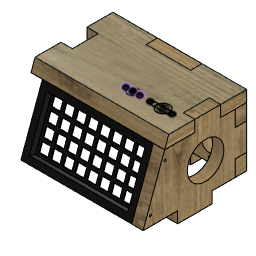
soundboard (Autodesk Fusion 360 design; units mm, degrees)
Autodesk Fusion 360 part; units mm, degrees
note: some values were not read from the file. Chosen so that the rebuilt part matches the saved one: which face or edge a step refers to. Set by a fixed rule: which sketch regions a step uses.
(part 1 of 2)
sketch "Skizze1" plane through (0, 0, 0) normal (1, 0, 0) x (0, 1, 0)
  line L0 (65, 65) -> (-65, 65)
  line L1 (-65, 65) -> (-65, -65)
  line L2 (-65, -65) -> (65, -65)
  line L3 (65, -65) -> (65, 65)
  line L4 (65, 65) -> (-65, -65) construction
  line L5 (-65, 65) -> (65, -65) construction
  circle A0 centre (0, 0) radius 29
  line L6 (65, 47) -> (-65, 47)
  line L7 (-65, -65) -> (-138, -65)
  line L8 (65, -47) -> (-138, -47)
  line L9 (-65, 47) -> (-99.2132, -47)
  line L10 (-65, 47) -> (35.0327, 47) construction
  line L11 (-99.2132, -47) -> (-99.2132, -65)
  line L12 (47, 65) -> (47, -65)
  dimension "d3" = 130
  dimension "d4" = 130
  dimension "d5" = 58
  dimension "d6" = 18
  dimension "d7" = 18
  dimension "d8" = 110
  dimension "d9" = 18
  constraint horizontal L0
  constraint perpendicular L0 L1
  constraint parallel L0 L2
  constraint parallel L1 L3
  constraint coincident L4 A0.centre
  constraint coincident L5 A0.centre
  constraint coincident A0.centre origin
  constraint coincident L3 L6.start
  constraint coincident L1 L6.end
  constraint perpendicular L1 L6
  constraint perpendicular L1 L7
  constraint coincident L3 L8.start
  constraint perpendicular L3 L8
  constraint horizontal L10
  constraint coincident L8 L9.end
  constraint coincident L7 L11.end
  constraint perpendicular L7 L11
  constraint coincident L0 L12.start
  constraint coincident L2 L12.end
  constraint perpendicular L2 L12
  measures "d3" distance of L1.end L2.end
  measures "d4" distance of L0.end L1.end
  measures "d5" diameter of A0
  measures "d6" distance of L0 L6
  measures "d7" distance of L7 L8
  measures "d8" angle of L9 L10
  measures "d9" distance of L3 L12
extrude "Extrusion1" add sketch "Skizze1" along normal blind 18 makes body 1
extrude "Extrusion2" add sketch "Skizze1" along normal blind 212.2 separate body contours L2 L3 L8 L12 | L1 L2 L8 L12 | L1 L7 L8 L11 makes body 2
extrude "Extrusion3" add sketch "Skizze1" along normal up to surface (212.2 mm away) separate body contours L0 L3 L6 L12 | L3 L6 L8 L12 | L2 L3 L8 L12 makes body 3
extrude "Extrusion4" add sketch "Skizze1" along normal up to surface (212.2 mm away) separate body contours L0 L3 L6 L12 | L0 L1 L6 L12 makes body 4
ref_plane "Arbeitsebene1" through (106.1, 0, 56) normal (1, 0, 0) x (0, 0, -1)
mirror "Spiegeln1" about plane through (106.1, 0, 56) normal (1, 0, 0) of bodies 1 makes body 5
ref_plane "Arbeitsebene2" through (18, -65, 47) normal (0, 0.939693, -0.34202) x (-1, 0, 0)
sketch "Skizze2" plane through (18, -65, 47) normal (0, 0.939693, -0.34202) x (-1, 0, 0)
  line L0 (18, 0) -> (-194.2, 0)
  line L1 (0, 0) -> (0, -100.0327)
  line L2 (18, -100.0327) -> (-194.2, -100.0327)
  line L3 (-176.2, 0) -> (-176.2, -100.0327)
  line L4 (18, -0.2) -> (-194.2, -0.2)
  line L5 (18, -99.8327) -> (-194.2, -99.8327)
  line L6 (-0.2, 0) -> (-0.2, -100.0327)
  line L7 (-176, 0) -> (-176, -100.0327)
  dimension "d22" = -0.2
  dimension "d23" = 0.2
  dimension "d24" = 0.2
  dimension "d25" = -0.2
ref_plane "Arbeitsebene3" through (106.1, -17.1066, 0) normal (-1, 0, 0) x (0, 1, 0)
sketch "Skizze3" plane through (106.1, -17.1066, 0) normal (-1, 0, 0) x (0, 1, 0)
  line L0 (-47.8934, -47) -> (-82.1066, 47)
  line L1 (-65, 0) -> (-52.8684, 0)
  line L2 (-65, 0) -> (-54.2875, 3.899) construction
  line L3 (-54.2875, 3.899) -> (-51.4492, -3.899) construction
  dimension "d73" = 11.4
  dimension "d74" = 12.1316
  dimension "d75" = 20
  dimension "d77" = 11.4
  constraint midpoint L0 L1.start
  constraint horizontal L1
  constraint perpendicular L0 L2
  constraint perpendicular L2 L3
  constraint midpoint L1.end L3
  measures "d73" distance of L1.start L2.end
  measures "d74" distance of L1.start L1.end
  measures "d75" angle of L1 L2
  measures "d77" distance of L1.start L2.end
sweep "Sweeping1" add profiles "Skizze2" path "Skizze3" along L1 section 1 contours L4 L5 L6 L7 separate body makes body 6
sketch "Skizze4" plane through (18, -65, 47) normal (0, 0.939693, -0.34202) x (-1, 0, 0)
  line L0 (-0.2, -0.2) -> (-0.2, -99.8327)
  line L1 (-0.2, -99.8327) -> (-176, -99.8327)
  line L2 (-176, -0.2) -> (-0.2, -0.2)
  line L3 (-14.6, -14.5158) -> (-28.6, -14.5158)
  line L4 (-28.6, -14.5158) -> (-28.6, -28.5158)
  line L5 (-28.6, -28.5158) -> (-14.6, -28.5158)
  line L6 (-14.6, -28.5158) -> (-14.6, -14.5158)
  line L7 (-33.6, -14.5158) -> (-47.6, -14.5158)
  line L8 (-33.6, -28.5158) -> (-33.6, -14.5158)
  line L9 (-47.6, -28.5158) -> (-33.6, -28.5158)
  line L10 (-47.6, -14.5158) -> (-47.6, -28.5158)
  line L11 (-52.6, -14.5158) -> (-66.6, -14.5158)
  line L12 (-52.6, -28.5158) -> (-52.6, -14.5158)
  line L13 (-66.6, -28.5158) -> (-52.6, -28.5158)
  line L14 (-66.6, -14.5158) -> (-66.6, -28.5158)
  line L15 (-71.6, -14.5158) -> (-85.6, -14.5158)
  line L16 (-71.6, -28.5158) -> (-71.6, -14.5158)
  line L17 (-85.6, -28.5158) -> (-71.6, -28.5158)
  line L18 (-85.6, -14.5158) -> (-85.6, -28.5158)
  line L19 (-90.6, -14.5158) -> (-104.6, -14.5158)
  line L20 (-90.6, -28.5158) -> (-90.6, -14.5158)
  line L21 (-104.6, -28.5158) -> (-90.6, -28.5158)
  line L22 (-104.6, -14.5158) -> (-104.6, -28.5158)
  line L23 (-109.6, -14.5158) -> (-123.6, -14.5158)
  line L24 (-109.6, -28.5158) -> (-109.6, -14.5158)
  line L25 (-123.6, -28.5158) -> (-109.6, -28.5158)
  line L26 (-123.6, -14.5158) -> (-123.6, -28.5158)
  line L27 (-128.6, -14.5158) -> (-142.6, -14.5158)
  line L28 (-128.6, -28.5158) -> (-128.6, -14.5158)
  line L29 (-142.6, -28.5158) -> (-128.6, -28.5158)
  line L30 (-142.6, -14.5158) -> (-142.6, -28.5158)
  line L31 (-147.6, -14.5158) -> (-161.6, -14.5158)
  line L32 (-147.6, -28.5158) -> (-147.6, -14.5158)
  line L33 (-161.6, -28.5158) -> (-147.6, -28.5158)
  line L34 (-161.6, -14.5158) -> (-161.6, -28.5158)
  line L35 (-14.6, -33.5158) -> (-28.6, -33.5158)
  line L36 (-14.6, -47.5158) -> (-14.6, -33.5158)
  line L37 (-28.6, -47.5158) -> (-14.6, -47.5158)
  line L38 (-28.6, -33.5158) -> (-28.6, -47.5158)
  line L39 (-33.6, -33.5158) -> (-47.6, -33.5158)
  line L40 (-33.6, -47.5158) -> (-33.6, -33.5158)
  line L41 (-47.6, -47.5158) -> (-33.6, -47.5158)
  line L42 (-47.6, -33.5158) -> (-47.6, -47.5158)
  line L43 (-52.6, -33.5158) -> (-66.6, -33.5158)
  line L44 (-52.6, -47.5158) -> (-52.6, -33.5158)
  line L45 (-66.6, -47.5158) -> (-52.6, -47.5158)
  line L46 (-66.6, -33.5158) -> (-66.6, -47.5158)
  line L47 (-71.6, -33.5158) -> (-85.6, -33.5158)
  line L48 (-71.6, -47.5158) -> (-71.6, -33.5158)
  line L49 (-85.6, -47.5158) -> (-71.6, -47.5158)
  line L50 (-85.6, -33.5158) -> (-85.6, -47.5158)
  line L51 (-90.6, -33.5158) -> (-104.6, -33.5158)
  line L52 (-90.6, -47.5158) -> (-90.6, -33.5158)
  line L53 (-104.6, -47.5158) -> (-90.6, -47.5158)
  line L54 (-104.6, -33.5158) -> (-104.6, -47.5158)
  line L55 (-109.6, -33.5158) -> (-123.6, -33.5158)
  line L56 (-109.6, -47.5158) -> (-109.6, -33.5158)
  line L57 (-123.6, -47.5158) -> (-109.6, -47.5158)
  line L58 (-123.6, -33.5158) -> (-123.6, -47.5158)
  line L59 (-128.6, -33.5158) -> (-142.6, -33.5158)
  line L60 (-128.6, -47.5158) -> (-128.6, -33.5158)
  line L61 (-142.6, -47.5158) -> (-128.6, -47.5158)
  line L62 (-142.6, -33.5158) -> (-142.6, -47.5158)
  line L63 (-147.6, -33.5158) -> (-161.6, -33.5158)
  line L64 (-147.6, -47.5158) -> (-147.6, -33.5158)
  line L65 (-161.6, -47.5158) -> (-147.6, -47.5158)
  line L66 (-161.6, -33.5158) -> (-161.6, -47.5158)
  line L67 (-14.6, -52.5158) -> (-28.6, -52.5158)
  line L68 (-14.6, -66.5158) -> (-14.6, -52.5158)
  line L69 (-28.6, -66.5158) -> (-14.6, -66.5158)
  line L70 (-28.6, -52.5158) -> (-28.6, -66.5158)
  line L71 (-33.6, -52.5158) -> (-47.6, -52.5158)
  line L72 (-33.6, -66.5158) -> (-33.6, -52.5158)
  line L73 (-47.6, -66.5158) -> (-33.6, -66.5158)
  line L74 (-47.6, -52.5158) -> (-47.6, -66.5158)
  line L75 (-52.6, -52.5158) -> (-66.6, -52.5158)
  line L76 (-52.6, -66.5158) -> (-52.6, -52.5158)
  line L77 (-66.6, -66.5158) -> (-52.6, -66.5158)
  line L78 (-66.6, -52.5158) -> (-66.6, -66.5158)
  line L79 (-71.6, -52.5158) -> (-85.6, -52.5158)
  line L80 (-71.6, -66.5158) -> (-71.6, -52.5158)
  line L81 (-85.6, -66.5158) -> (-71.6, -66.5158)
  line L82 (-85.6, -52.5158) -> (-85.6, -66.5158)
  line L83 (-90.6, -52.5158) -> (-104.6, -52.5158)
  line L84 (-90.6, -66.5158) -> (-90.6, -52.5158)
  line L85 (-104.6, -66.5158) -> (-90.6, -66.5158)
  line L86 (-104.6, -52.5158) -> (-104.6, -66.5158)
  line L87 (-109.6, -52.5158) -> (-123.6, -52.5158)
  line L88 (-109.6, -66.5158) -> (-109.6, -52.5158)
  line L89 (-123.6, -66.5158) -> (-109.6, -66.5158)
  line L90 (-123.6, -52.5158) -> (-123.6, -66.5158)
  line L91 (-128.6, -52.5158) -> (-142.6, -52.5158)
  line L92 (-128.6, -66.5158) -> (-128.6, -52.5158)
  line L93 (-142.6, -66.5158) -> (-128.6, -66.5158)
  line L94 (-142.6, -52.5158) -> (-142.6, -66.5158)
  line L95 (-147.6, -52.5158) -> (-161.6, -52.5158)
  line L96 (-147.6, -66.5158) -> (-147.6, -52.5158)
  line L97 (-161.6, -66.5158) -> (-147.6, -66.5158)
  line L98 (-161.6, -52.5158) -> (-161.6, -66.5158)
  line L99 (-14.6, -71.5158) -> (-28.6, -71.5158)
  line L100 (-14.6, -85.5158) -> (-14.6, -71.5158)
  line L101 (-28.6, -85.5158) -> (-14.6, -85.5158)
  line L102 (-28.6, -71.5158) -> (-28.6, -85.5158)
  line L103 (-33.6, -71.5158) -> (-47.6, -71.5158)
  line L104 (-33.6, -85.5158) -> (-33.6, -71.5158)
  line L105 (-47.6, -85.5158) -> (-33.6, -85.5158)
  line L106 (-47.6, -71.5158) -> (-47.6, -85.5158)
  line L107 (-52.6, -71.5158) -> (-66.6, -71.5158)
  line L108 (-52.6, -85.5158) -> (-52.6, -71.5158)
  line L109 (-66.6, -85.5158) -> (-52.6, -85.5158)
  line L110 (-66.6, -71.5158) -> (-66.6, -85.5158)
  line L111 (-71.6, -71.5158) -> (-85.6, -71.5158)
  line L112 (-71.6, -85.5158) -> (-71.6, -71.5158)
  line L113 (-85.6, -85.5158) -> (-71.6, -85.5158)
  line L114 (-85.6, -71.5158) -> (-85.6, -85.5158)
  line L115 (-90.6, -71.5158) -> (-104.6, -71.5158)
  line L116 (-90.6, -85.5158) -> (-90.6, -71.5158)
  line L117 (-104.6, -85.5158) -> (-90.6, -85.5158)
  line L118 (-104.6, -71.5158) -> (-104.6, -85.5158)
  line L119 (-109.6, -71.5158) -> (-123.6, -71.5158)
  line L120 (-109.6, -85.5158) -> (-109.6, -71.5158)
  line L121 (-123.6, -85.5158) -> (-109.6, -85.5158)
  line L122 (-123.6, -71.5158) -> (-123.6, -85.5158)
  line L123 (-128.6, -71.5158) -> (-142.6, -71.5158)
  line L124 (-128.6, -85.5158) -> (-128.6, -71.5158)
  line L125 (-142.6, -85.5158) -> (-128.6, -85.5158)
  line L126 (-142.6, -71.5158) -> (-142.6, -85.5158)
  line L127 (-147.6, -71.5158) -> (-161.6, -71.5158)
  line L128 (-147.6, -85.5158) -> (-147.6, -71.5158)
  line L129 (-161.6, -85.5158) -> (-147.6, -85.5158)
  line L130 (-161.6, -71.5158) -> (-161.6, -85.5158)
  line L131 (-0.2, 0) -> (-0.2, -100.0327)
  line L132 (-161.6, -85.5158) -> (-14.6, -14.5158) construction
  line L133 (-161.6, -14.5158) -> (-14.6, -85.5158) construction
  line L134 (18, -99.8327) -> (-194.2, -99.8327)
  line L135 (18, -0.2) -> (-194.2, -0.2)
  line L136 (-10.2, -89.8327) -> (-166.2, -89.8327)
  line L137 (-166.2, -89.8327) -> (-166.2, -10.2)
  line L138 (-166.2, -10.2) -> (-10.2, -10.2)
  line L139 (-10.2, -10.2) -> (-10.2, -89.8327)
  line L140 (-176, -99.8327) -> (-176, -0.2)
  point P0 (-88.1, -0.2)
  point P1 (-176.2, -50.0158)
  point P2 (-88.1, -50.0158)
  dimension "d33" = 14
  dimension "d34" = 14
  dimension "d37" = -19
  dimension "d38" = -19
  dimension "d41" = 14.5
  dimension "d42" = 14.3164
  dimension "d43" = 14.3164
  dimension "d52" = 14.4
  constraint horizontal L3
  constraint vertical L4
  constraint horizontal L5
  constraint vertical L6
  constraint midpoint L2 P0
  constraint midpoint L133 P2
  constraint horizontal P1 P2
  constraint vertical P0 P2
  constraint parallel L1 L136
  constraint parallel L2 L138
  constraint parallel L0 L139
  measures "d33" distance of L3.start L3.end
  measures "d34" distance of L3.start L5.end
  measures "d52" distance of L34 L140
sketch "Skizze5" plane through (106.1, -17.1066, 0) normal (-1, 0, 0) x (0, 1, 0)
  line L0 (-65, 0) -> (-52.8684, 0)
  line L1 (-65, 0) -> (-54.3582, 0)
  line L2 (-54.2875, 3.899) -> (-51.4492, -3.899)
  line L3 (-65, 0) -> (-54.2875, 3.899)
  line L4 (-55.6031, 3.4202) -> (-65, 0)
  point P0 (-52.8684, 0)
  point P1 (-55.6031, 3.4202)
  dimension "d76" = 1.4
  dimension "d79" = 1.4
  constraint coincident L0.start L1.start
  constraint coincident L0 L1.end
  constraint parallel L0 L1
  constraint coincident L3 P1
  constraint coincident P1 L4.start
  measures "d76" distance of L1.end L2
  measures "d79" distance of L2.start P1
sweep "Sweeping3" cut kept parallel profiles "Skizze4" path "Skizze5" along L4 section 1 contours L3 L4 L5 L6 | L7 L8 L9 L10 | L11 L12 L13 L14 | L15 L16 L17 L18 | L19 L20 L21 L22 | L23 L24 L25 L26 | L27 L28 L29 L30 | L31 L32 L33 L34 | L35 L36 L37 L38 | L39 L40 L41 L42 | L43 L44 L45 L46 | L47 L48 L49 L50 | L51 L52 L53 L54 | L55 L56 L57 L58 | L59 L60 L61 L62 | L63 L64 L65 L66 | L67 L68 L69 L70 | L71 L72 L73 L74 | L75 L76 L77 L78 | L79 L80 L81 L82 | L83 L84 L85 L86 | L87 L88 L89 L90 | L91 L92 L93 L94 | L95 L96 L97 L98 | L99 L100 L101 L102 | L103 L104 L105 L106 | L107 L108 L109 L110 | L111 L112 L113 L114 | L115 L116 L117 L118 | L119 L120 L121 L122 | L123 L124 L125 L126 | L127 L128 L129 L130 | L136 L137 L138 L139 bodies 6
sketch "Skizze6" plane through (0, -63.105, 22.9684) normal (0, -0.939693, 0.34202) x (1, 0, 0)
  line L0 (184.2, 14.4704) -> (28.2, 14.4704)
  line L1 (28.2, 14.4704) -> (28.2, -65.1623)
  line L2 (28.2, -65.1623) -> (184.2, -65.1623)
  line L3 (184.2, -65.1623) -> (184.2, 14.4704)
  line L4 (165.6, -6.5816) -> (165.6, 7.4184)
  line L5 (165.6, 7.4184) -> (179.6, 7.4184)
  line L6 (179.6, 7.4184) -> (179.6, -6.5816)
  line L7 (179.6, -6.5816) -> (165.6, -6.5816)
  line L8 (165.6, -11.5816) -> (179.6, -11.5816)
  line L9 (165.6, -25.5816) -> (165.6, -11.5816)
  line L10 (179.6, -25.5816) -> (165.6, -25.5816)
  line L11 (179.6, -11.5816) -> (179.6, -25.5816)
  line L12 (165.6, -30.5816) -> (179.6, -30.5816)
  line L13 (165.6, -44.5816) -> (165.6, -30.5816)
  line L14 (179.6, -44.5816) -> (165.6, -44.5816)
  line L15 (179.6, -30.5816) -> (179.6, -44.5816)
  line L16 (165.6, -49.5816) -> (179.6, -49.5816)
  line L17 (165.6, -63.5816) -> (165.6, -49.5816)
  line L18 (179.6, -63.5816) -> (165.6, -63.5816)
  line L19 (179.6, -49.5816) -> (179.6, -63.5816)
  line L20 (146.6, 7.4184) -> (160.6, 7.4184)
  line L21 (146.6, -6.5816) -> (146.6, 7.4184)
  line L22 (160.6, -6.5816) -> (146.6, -6.5816)
  line L23 (160.6, 7.4184) -> (160.6, -6.5816)
  line L24 (146.6, -11.5816) -> (160.6, -11.5816)
  line L25 (146.6, -25.5816) -> (146.6, -11.5816)
  line L26 (160.6, -25.5816) -> (146.6, -25.5816)
  line L27 (160.6, -11.5816) -> (160.6, -25.5816)
  line L28 (146.6, -30.5816) -> (160.6, -30.5816)
  line L29 (146.6, -44.5816) -> (146.6, -30.5816)
  line L30 (160.6, -44.5816) -> (146.6, -44.5816)
  line L31 (160.6, -30.5816) -> (160.6, -44.5816)
  line L32 (146.6, -49.5816) -> (160.6, -49.5816)
  line L33 (146.6, -63.5816) -> (146.6, -49.5816)
  line L34 (160.6, -63.5816) -> (146.6, -63.5816)
  line L35 (160.6, -49.5816) -> (160.6, -63.5816)
  line L36 (141.6, -49.5816) -> (141.6, -63.5816)
  line L37 (127.6, -49.5816) -> (141.6, -49.5816)
  line L38 (127.6, -63.5816) -> (127.6, -49.5816)
  line L39 (141.6, -63.5816) -> (127.6, -63.5816)
  line L40 (127.6, -30.5816) -> (141.6, -30.5816)
  line L41 (127.6, -44.5816) -> (127.6, -30.5816)
  line L42 (141.6, -44.5816) -> (127.6, -44.5816)
  line L43 (141.6, -30.5816) -> (141.6, -44.5816)
  line L44 (141.6, -25.5816) -> (127.6, -25.5816)
  line L45 (141.6, -11.5816) -> (141.6, -25.5816)
  line L46 (127.6, -11.5816) -> (141.6, -11.5816)
  line L47 (127.6, -25.5816) -> (127.6, -11.5816)
  line L48 (141.6, 7.4184) -> (141.6, -6.5816)
  line L49 (127.6, 7.4184) -> (141.6, 7.4184)
  line L50 (127.6, -6.5816) -> (127.6, 7.4184)
  line L51 (141.6, -6.5816) -> (127.6, -6.5816)
  line L52 (122.6, -6.5816) -> (108.6, -6.5816)
  line L53 (108.6, -6.5816) -> (108.6, 7.4184)
  line L54 (108.6, 7.4184) -> (122.6, 7.4184)
  line L55 (122.6, 7.4184) -> (122.6, -6.5816)
  line L56 (89.6, 7.4184) -> (103.6, 7.4184)
  line L57 (89.6, -6.5816) -> (89.6, 7.4184)
  line L58 (103.6, -6.5816) -> (89.6, -6.5816)
  line L59 (103.6, 7.4184) -> (103.6, -6.5816)
  line L60 (103.6, -44.5816) -> (89.6, -44.5816)
  line L61 (89.6, -44.5816) -> (89.6, -30.5816)
  line L62 (89.6, -30.5816) -> (103.6, -30.5816)
  line L63 (103.6, -30.5816) -> (103.6, -44.5816)
  line L64 (103.6, -25.5816) -> (89.6, -25.5816)
  line L65 (89.6, -25.5816) -> (89.6, -11.5816)
  line L66 (89.6, -11.5816) -> (103.6, -11.5816)
  line L67 (103.6, -11.5816) -> (103.6, -25.5816)
  line L68 (108.6, -11.5816) -> (122.6, -11.5816)
  line L69 (108.6, -25.5816) -> (108.6, -11.5816)
  line L70 (122.6, -25.5816) -> (108.6, -25.5816)
  line L71 (122.6, -11.5816) -> (122.6, -25.5816)
  line L72 (122.6, -44.5816) -> (108.6, -44.5816)
  line L73 (108.6, -44.5816) -> (108.6, -30.5816)
  line L74 (108.6, -30.5816) -> (122.6, -30.5816)
  line L75 (108.6, -49.5816) -> (122.6, -49.5816)
  line L76 (108.6, -63.5816) -> (108.6, -49.5816)
  line L77 (122.6, -63.5816) -> (108.6, -63.5816)
  line L78 (122.6, -49.5816) -> (122.6, -63.5816)
  line L79 (89.6, -49.5816) -> (103.6, -49.5816)
  line L80 (89.6, -63.5816) -> (89.6, -49.5816)
  line L81 (103.6, -63.5816) -> (89.6, -63.5816)
  line L82 (103.6, -49.5816) -> (103.6, -63.5816)
  line L83 (70.6, -49.5816) -> (84.6, -49.5816)
  line L84 (70.6, -63.5816) -> (70.6, -49.5816)
  line L85 (84.6, -63.5816) -> (70.6, -63.5816)
  line L86 (84.6, -49.5816) -> (84.6, -63.5816)
  line L87 (84.6, -30.5816) -> (84.6, -44.5816)
  line L88 (70.6, -30.5816) -> (84.6, -30.5816)
  line L89 (70.6, -44.5816) -> (70.6, -30.5816)
  line L90 (84.6, -44.5816) -> (70.6, -44.5816)
  line L91 (70.6, -25.5816) -> (70.6, -11.5816)
  line L92 (70.6, -11.5816) -> (84.6, -11.5816)
  line L93 (84.6, -11.5816) -> (84.6, -25.5816)
  line L94 (84.6, -25.5816) -> (70.6, -25.5816)
  line L95 (70.6, -6.5816) -> (70.6, 7.4184)
  line L96 (70.6, 7.4184) -> (84.6, 7.4184)
  line L97 (84.6, 7.4184) -> (84.6, -6.5816)
  line L98 (84.6, -6.5816) -> (70.6, -6.5816)
  line L99 (51.6, 7.4184) -> (65.6, 7.4184)
  line L100 (51.6, -6.5816) -> (51.6, 7.4184)
  line L101 (65.6, -6.5816) -> (51.6, -6.5816)
  line L102 (65.6, 7.4184) -> (65.6, -6.5816)
  line L103 (51.6, -11.5816) -> (65.6, -11.5816)
  line L104 (51.6, -25.5816) -> (51.6, -11.5816)
  line L105 (65.6, -25.5816) -> (51.6, -25.5816)
  line L106 (65.6, -11.5816) -> (65.6, -25.5816)
  line L107 (51.6, -30.5816) -> (65.6, -30.5816)
  line L108 (51.6, -44.5816) -> (51.6, -30.5816)
  line L109 (65.6, -44.5816) -> (51.6, -44.5816)
  line L110 (65.6, -30.5816) -> (65.6, -44.5816)
  line L111 (51.6, -49.5816) -> (65.6, -49.5816)
  line L112 (51.6, -63.5816) -> (51.6, -49.5816)
  line L113 (65.6, -63.5816) -> (51.6, -63.5816)
  line L114 (65.6, -49.5816) -> (65.6, -63.5816)
  line L115 (32.6, 7.4184) -> (46.6, 7.4184)
  line L116 (32.6, -6.5816) -> (32.6, 7.4184)
  line L117 (46.6, -6.5816) -> (32.6, -6.5816)
  line L118 (46.6, 7.4184) -> (46.6, -6.5816)
  line L119 (32.6, -11.5816) -> (46.6, -11.5816)
  line L120 (32.6, -25.5816) -> (32.6, -11.5816)
  line L121 (46.6, -25.5816) -> (32.6, -25.5816)
  line L122 (46.6, -11.5816) -> (46.6, -25.5816)
  line L123 (32.6, -30.5816) -> (46.6, -30.5816)
  line L124 (32.6, -44.5816) -> (32.6, -30.5816)
  line L125 (46.6, -44.5816) -> (32.6, -44.5816)
  line L126 (46.6, -30.5816) -> (46.6, -44.5816)
  line L127 (32.6, -49.5816) -> (46.6, -49.5816)
  line L128 (32.6, -63.5816) -> (32.6, -49.5816)
  line L129 (46.6, -63.5816) -> (32.6, -63.5816)
  line L130 (46.6, -49.5816) -> (46.6, -63.5816)
  line L131 (122.6, -30.5816) -> (122.6, -44.5816)
  line L132 (28.2, 11.7342) -> (28.2, -67.8985)
  line L133 (28.2, -67.8985) -> (184.2, -67.8985)
  line L134 (184.2, -67.8985) -> (184.2, 11.7342)
  line L135 (184.2, 11.7342) -> (28.2, 11.7342)
  line L136 (184.2, 11.7342) -> (28.2, 11.7342)
  line L137 (28.2, 11.7342) -> (28.2, -67.8985)
  line L138 (28.2, -67.8985) -> (184.2, -67.8985)
  line L139 (184.2, -67.8985) -> (184.2, 11.7342)
extrude "Extrusion5" cut sketch "Skizze6" against normal up to surface (1.4 mm away) contours L4 L5 L6 L7 | L8 L9 L10 L11 | L12 L13 L14 L15 | L16 L17 L18 L19 | L20 L21 L22 L23 | L24 L25 L26 L27 | L28 L29 L30 L31 | L32 L33 L34 L35 | L36 L37 L38 L39 | L40 L41 L42 L43 | L44 L45 L46 L47 | L48 L49 L50 L51 | L52 L53 L54 L55 | L56 L57 L58 L59 | L60 L61 L62 L63 | L64 L65 L66 L67 | L68 L69 L70 L71 | L72 L73 L74 L131 | L75 L76 L77 L78 | L79 L80 L81 L82 | L83 L84 L85 L86 | L87 L88 L89 L90 | L91 L92 L93 L94 | L95 L96 L97 L98 | L99 L100 L101 L102 | L103 L104 L105 L106 | L107 L108 L109 L110 | L111 L112 L113 L114 | L115 L116 L117 L118 | L119 L120 L121 L122 | L123 L124 L125 L126 | L127 L128 L129 L130 bodies 6
sketch "Skizze7" plane through (0, 0, 0) normal (1, 0, 0) x (0, 1, 0)
  line L0 (-65, 47) -> (-99.2132, -47)
  line L1 (-65, 65) -> (65, 65)
  line L2 (65, 65) -> (65, 47)
  line L3 (65, 47) -> (-65, 47)
  line L4 (-65, 47) -> (-65, 65)
  line L5 (-65, 47) -> (-58.4485, 65)
  line L6 (-58.4485, 65) -> (-65, 65)
  line L7 (-65, 65) -> (-65, 47)
  constraint coincident L0.start L3.end
  constraint coincident L1 L5.end
  constraint parallel L0 L5
  constraint coincident L1.start L4.end
extrude "Extrusion6" cut sketch "Skizze7" along normal up to surface (212.2 mm away) contours L1 L4 L5 L6 L7 bodies 1 4 5
sketch "Skizze8" plane through (194, 0, 0) normal (1, 0, 0) x (0, 1, 0)
  line L0 (-65.0684, 46.8121) -> (-99.1448, -46.8121)
  line L1 (-99.1448, -46.8121) -> (-87.0132, -46.8121)
  line L2 (-87.0132, -46.8121) -> (-52.9368, 46.8121)
  line L3 (-52.9368, 46.8121) -> (-65.0684, 46.8121)
  line L4 (-69.75, 33.9495) -> (-59.0375, 30.0505) construction
  line L5 (-93.0441, -30.0505) -> (-82.3316, -33.9495) construction
  line L6 (-64.3937, 32) -> (-87.6878, -32) construction
  line L7 (65, -47) -> (-99.2132, -47) construction
  line L8 (65, 47) -> (-65, 47) construction
  circle A0 centre (-64.3937, 32) radius 2
  circle A1 centre (-87.6878, -32) radius 2
  point P0 (-64.3937, 32)
  point P1 (-87.6878, -32)
  dimension "d59" = 15
  dimension "d60" = 15
  dimension "d61" = 4
  dimension "d62" = 4
  constraint coincident L0 L4.start
  constraint coincident L2 L4.end
  constraint perpendicular L2 L4
  constraint coincident L0 L5.start
  constraint coincident L2 L5.end
  constraint perpendicular L2 L5
  constraint midpoint L4 P0
  constraint midpoint L5 P1
  constraint coincident P0 L6.start
  constraint coincident P1 L6.end
  measures "d59" distance of P1 L7
  measures "d60" distance of P0 L8
  measures "d61" diameter of A0
  measures "d62" diameter of A1
extrude "Extrusion8" add sketch "Skizze8" against normal blind 7 separate body contours A0 | A1 makes body 7 at (189.3333, -65.7902, 33.4317) makes body 8 at (189.3333, -85.6978, -32.1991)
mirror "Spiegeln2" about plane through (106.1, 0, 56) normal (1, 0, 0) of bodies 7 8 makes body 9 at (22.8667, -65.7902, 33.4317) makes body 10 at (22.8667, -85.6978, -32.1991)
combine "Kombinieren1" operation cut target body 6 tool bodies 9 10 7 8
sketch "Skizze9" plane through (212.2, 0, 0) normal (1, 0, 0) x (0, 1, 0)
  line L0 (-58.4485, 65) -> (-99.2132, -47)
  line L1 (-99.2132, -47) -> (-99.2132, -65)
  line L2 (-99.2132, -65) -> (65, -65)
  line L3 (65, -65) -> (65, 65)
  circle A0 centre (0, 0) radius 29
  circle A1 centre (-64.3937, 32) radius 1.75
  circle A2 centre (-87.6878, -32) radius 1.75
  line L4 (65, 65) -> (-58.4485, 65)
  point P0 (-64.3937, 32)
  point P1 (-87.6878, -32)
  dimension "d67" = 3.5
  dimension "d68" = 3.5
  constraint coincident P0 A1.centre
  constraint coincident P1 A2.centre
  measures "d67" diameter of A1
  measures "d68" diameter of A2
extrude "Extrusion9" add sketch "Skizze9" against normal up to surface (18.2 mm away) separate body contours A1 | A2 makes body 11 at (200.0667, -65.6157, 33.2528) makes body 12 at (200.0667, -88.7094, -33.4209)
mirror "Spiegeln3" about plane through (106.1, 0, 56) normal (1, 0, 0) of bodies 11 12 makes body 13 at (12.1333, -65.6157, 33.2528) makes body 14 at (12.1333, -88.7094, -33.4209)
combine "Kombinieren2" operation cut target body 5 tool bodies 11 12
combine "Kombinieren3" operation cut target body 1 tool bodies 13 14
sketch "Skizze14" plane through (0, 0, 65) normal (0, 0, 1) x (-1, 0, 0)
  line L0 (0, 58.4485) -> (-212.2, 58.4485)
  line L1 (-212.2, 58.4485) -> (-212.2, -65)
  line L2 (-212.2, -65) -> (0, -65)
  line L3 (0, -65) -> (0, 58.4485)
  line L4 (-212.2, 58.4485) -> (-194.2, 58.4485)
  line L5 (-194.2, 58.4485) -> (-194.2, 17.299)
  line L6 (-194.2, 17.299) -> (-212.2, 17.299)
  line L7 (-212.2, 17.299) -> (-212.2, 58.4485)
  line L8 (-212.2, -65) -> (-194.2, -65)
  line L9 (-194.2, -65) -> (-194.2, -23.8505)
  line L10 (-194.2, -23.8505) -> (-212.2, -23.8505)
  line L11 (-212.2, -23.8505) -> (-212.2, -65)
  line L12 (-194.2, 58.4485) -> (-212.2, 58.4485)
  line L13 (-212.2, 58.4485) -> (-212.2, -65)
  line L14 (-212.2, -65) -> (-194.2, -65)
  line L15 (-194.2, -65) -> (-194.2, 58.4485)
  line L16 (-212.2, 99.2132) -> (-212.2, 58.4485)
  line L17 (-212.2, 58.4485) -> (-194.2, 58.4485)
  line L18 (-194.2, 58.4485) -> (-194.2, 99.2132)
  line L19 (-194.2, 99.2132) -> (-212.2, 99.2132)
  dimension "d116" = 123.4485
  dimension "d117" = 18
  dimension "d118" = 41.1495
  dimension "d119" = 18
  dimension "d120" = 41.1495
  constraint horizontal L4
  constraint vertical L5
  constraint horizontal L6
  constraint vertical L7
  constraint coincident L0.end L1.start
  constraint horizontal L8
  constraint vertical L9
  constraint horizontal L10
  constraint vertical L11
  constraint coincident L1.end L2.start
  measures "d116" distance of L0.end L1.end
  measures "d117" distance of L0.end L4.end
  measures "d118" distance of L0.end L6.end
  measures "d119" distance of L1.end L8.end
  measures "d120" distance of L1.end L10.end
extrude "Extrusion21" cut sketch "Skizze14" against normal blind 18 contours L0 L1 L4 L5 L6 L7 L12 L13 L15 L17 | L0 L4 L12 L16 L17 L18 L19 | L1 L2 L8 L9 L10 L11 L13 L14 L15 bodies 5
extrude "Extrusion22" cut sketch "Skizze14" against normal blind 18 contours L1 L6 L10 L13 L15 bodies 4
sketch "Skizze15" plane through (0, 0, 65) normal (0, 0, 1) x (-1, 0, 0)
  line L0 (0, 58.4485) -> (-18, 58.4485)
  line L1 (-18, 58.4485) -> (-18, -65)
  line L2 (-18, -65) -> (0, -65)
  line L3 (0, -65) -> (0, 58.4485)
  line L4 (0, -65) -> (0, 58.4485)
  line L5 (0, -65) -> (-18, -65)
  line L6 (-18, -65) -> (-18, -23.8505)
  line L7 (-18, -23.8505) -> (0, -23.8505)
  line L8 (0, -23.8505) -> (0, -65)
  line L9 (-18, 58.4485) -> (0, 58.4485)
  line L10 (0, 58.4485) -> (0, 17.299)
  line L11 (0, 17.299) -> (-18, 17.299)
  line L12 (-18, 17.299) -> (-18, 58.4485)
  line L13 (0, 58.4485) -> (0, 99.2132)
  line L14 (0, 99.2132) -> (-18, 99.2132)
  line L15 (-18, 99.2132) -> (-18, 58.4485)
  line L16 (-18, 58.4485) -> (0, 58.4485)
  dimension "d131" = 123.4485
  dimension "d132" = 41.1495
  dimension "d133" = 41.1495
  constraint horizontal L5
  constraint vertical L6
  constraint horizontal L7
  constraint vertical L8
  constraint coincident L1 L6.end
  constraint coincident L2.end L3.start
  constraint horizontal L9
  constraint vertical L10
  constraint horizontal L11
  constraint vertical L12
  constraint coincident L0.end L1.start
  measures "d131" distance of L2.end L0.start
  measures "d132" distance of L2.end L7.end
  measures "d133" distance of L0.end L11.end
extrude "Extrusion23" cut sketch "Skizze15" against normal blind 18 contours L0 L1 L3 L4 L9 L10 L11 L12 L16 | L0 L9 L13 L14 L15 L16 | L1 L2 L3 L4 L5 L6 L7 L8 bodies 1
extrude "Extrusion24" cut sketch "Skizze15" against normal blind 18 contours L1 L3 L4 L7 L11 bodies 4
sketch "Skizze16" plane through (0, 0, -65) normal (0, 0, -1) x (1, 0, 0)
  line L0 (212.2, -65) -> (212.2, 99.2132)
  line L1 (212.2, 99.2132) -> (194.2, 99.2132)
  line L2 (194.2, 99.2132) -> (194.2, -65)
  line L3 (194.2, -65) -> (212.2, -65)
  line L4 (194.2, 99.2132) -> (212.2, 99.2132)
  line L5 (212.2, 99.2132) -> (212.2, 44.4755)
  line L6 (212.2, 44.4755) -> (194.2, 44.4755)
  line L7 (194.2, 44.4755) -> (194.2, 99.2132)
  line L8 (212.2, -65) -> (194.2, -65)
  line L9 (194.2, -65) -> (194.2, -10.2623)
  line L10 (194.2, -10.2623) -> (212.2, -10.2623)
  line L11 (212.2, -10.2623) -> (212.2, -65)
  dimension "d138" = 164.2132
  dimension "d139" = 54.7377
  dimension "d140" = 54.7377
  constraint horizontal L4
  constraint vertical L5
  constraint horizontal L6
  constraint vertical L7
  constraint coincident L0 L5.end
  constraint coincident L1.end L2.start
  constraint horizontal L8
  constraint vertical L9
  constraint horizontal L10
  constraint vertical L11
  constraint coincident L0.start L3.end
  measures "d138" distance of L1.end L2.end
  measures "d139" distance of L0.end L5.end
  measures "d140" distance of L0.start L10.end
extrude "Extrusion25" cut sketch "Skizze16" against normal blind 18 contours L0 L2 L3 L8 L9 L10 L11 | L0 L1 L2 L4 L5 L6 L7 bodies 5
extrude "Extrusion26" cut sketch "Skizze16" against normal blind 18 contours L0 L2 L6 L10 bodies 2
sketch "Skizze17" plane through (0, 0, -65) normal (0, 0, -1) x (1, 0, 0)
  line L0 (0, 99.2132) -> (0, -65)
  line L1 (0, -65) -> (18, -65)
  line L2 (18, -65) -> (18, 99.2132)
  line L3 (18, 99.2132) -> (0, 99.2132)
  line L4 (0, 99.2132) -> (18, 99.2132)
  line L5 (18, 99.2132) -> (18, 44.4755)
  line L6 (18, 44.4755) -> (0, 44.4755)
  line L7 (0, 44.4755) -> (0, 99.2132)
  line L8 (18, -65) -> (0, -65)
  line L9 (0, -65) -> (0, -10.2623)
  line L10 (0, -10.2623) -> (18, -10.2623)
  line L11 (18, -10.2623) -> (18, -65)
  dimension "d145" = 164.2132
  dimension "d146" = 54.7377
  dimension "d147" = 54.7377
  constraint horizontal L4
  constraint vertical L5
  constraint horizontal L6
  constraint vertical L7
  constraint coincident L2 L5.end
  constraint coincident L0.start L3.end
  constraint horizontal L8
  constraint vertical L9
  constraint horizontal L10
  constraint vertical L11
  constraint coincident L0 L9.end
  constraint coincident L1.end L2.start
  measures "d145" distance of L1.end L2.end
  measures "d146" distance of L0.start L6.end
  measures "d147" distance of L0.end L9.end
extrude "Extrusion27" cut sketch "Skizze17" against normal blind 18 contours L0 L2 L6 L10 bodies 2
extrude "Extrusion28" cut sketch "Skizze17" against normal blind 18 contours L0 L2 L3 L4 L5 L6 L7 | L0 L1 L2 L8 L9 L10 L11 bodies 1
sketch "Skizze18" plane through (0, 0, 65) normal (0, 0, 1) x (-1, 0, 0)
  line L0 (-212.2, -47) -> (-212.2, -65)
  line L1 (-212.2, -65) -> (0, -65)
  line L2 (0, -65) -> (0, -47)
  line L3 (0, -47) -> (-212.2, -47)
  line L4 (0, -65) -> (-70.7333, -65)
  line L5 (-70.7333, -65) -> (-70.7333, -47)
  line L6 (-70.7333, -47) -> (0, -47)
  line L7 (0, -47) -> (0, -65)
  line L8 (-212.2, -65) -> (-141.4667, -65)
  line L9 (-141.4667, -65) -> (-141.4667, -47)
  line L10 (-141.4667, -47) -> (-212.2, -47)
  line L11 (-212.2, -47) -> (-212.2, -65)
  dimension "d152" = 212.2
  dimension "d153" = 70.7333
  dimension "d154" = 70.7333
  constraint horizontal L4
  constraint vertical L5
  constraint horizontal L6
  constraint vertical L7
  constraint coincident L3 L5.end
  constraint coincident L1.end L2.start
  constraint horizontal L8
  constraint vertical L9
  constraint horizontal L10
  constraint vertical L11
  constraint coincident L3 L9.end
  constraint coincident L0.end L1.start
  measures "d152" distance of L0.end L1.end
  measures "d153" distance of L1.end L4.end
  measures "d154" distance of L0.end L8.end
extrude "Extrusion29" cut sketch "Skizze18" against normal blind 18 contours L1 L3 L5 L9 bodies 4
extrude "Extrusion30" cut sketch "Skizze18" against normal blind 18 contours L0 L1 L3 L8 L9 L10 L11 | L1 L2 L3 L4 L5 L6 L7 bodies 3
sketch "Skizze19" plane through (0, 0, -65) normal (0, 0, -1) x (1, 0, 0)
  line L0 (212.2, -65) -> (212.2, -47)
  line L1 (212.2, -47) -> (0, -47)
  line L2 (0, -47) -> (0, -65)
  line L3 (0, -65) -> (212.2, -65)
  line L4 (70.7333, -65) -> (70.7333, -47)
  line L5 (141.4667, -65) -> (141.4667, -47)
  line L6 (0, -47) -> (212.2, -47)
extrude "Extrusion31" cut sketch "Skizze19" against normal blind 18 contours L0 L1 L3 L5 L6 | L1 L2 L3 L4 L6 bodies 3
extrude "Extrusion32" cut sketch "Skizze19" against normal blind 18 contours L1 L3 L4 L5 L6 bodies 2
sketch "Skizze20" plane through (212.2, 0, 0) normal (1, 0, 0) x (0, 1, 0)
  line L0 (47, -47) -> (65, -47)
  line L1 (65, -47) -> (65, 47)
  line L2 (65, 47) -> (47, 47)
  line L3 (47, 47) -> (47, -47)
  line L4 (47, 65) -> (65, 65)
  line L5 (10.2623, -65) -> (65, -65)
  line L6 (65, 65) -> (47, 65)
  line L7 (47, 65) -> (47, 21.6667)
  line L8 (47, 21.6667) -> (65, 21.6667)
  line L9 (65, 21.6667) -> (65, 65)
  line L10 (65, -65) -> (47, -65)
  line L11 (47, -65) -> (47, -21.6667)
  line L12 (47, -21.6667) -> (65, -21.6667)
  line L13 (65, -21.6667) -> (65, -65)
  line L14 (47, -47) -> (47, 47)
  line L15 (65, -47) -> (65, 47)
  dimension "d163" = 130
  dimension "d164" = 43.3333
  dimension "d165" = 43.3333
  constraint horizontal L6
  constraint vertical L7
  constraint horizontal L8
  constraint vertical L9
  constraint coincident L3 L7.end
  constraint coincident L4.end L6.start
  constraint horizontal L10
  constraint vertical L11
  constraint horizontal L12
  constraint vertical L13
  constraint coincident L3 L11.end
  constraint coincident L5.end L10.start
  measures "d163" distance of L4 L5
  measures "d164" distance of L4.end L8.end
  measures "d165" distance of L5.end L12.end
extrude "Extrusion33" cut sketch "Skizze20" against normal blind 18 contours L0 L1 L3 L11 L12 L13 L14 L15 | L0 L5 L10 L11 L13 | L1 L2 L3 L7 L8 L9 L14 L15 | L2 L4 L6 L7 L9 bodies 5
extrude "Extrusion35" cut sketch "Skizze20" against normal blind 18 contours L0 L5 L10 L11 L13 | L1 L3 L8 L12 L14 L15 | L2 L4 L6 L7 L9 bodies 3
sketch "Skizze21" plane through (0, 0, 0) normal (-1, 0, 0) x (0, -1, 0)
  line L0 (-65, -47) -> (-47, -47)
  line L1 (-47, -47) -> (-47, 47)
  line L2 (-47, 47) -> (-65, 47)
  line L3 (-65, 47) -> (-65, -47)
  line L4 (-47, 21.6667) -> (-65, 21.6667)
  line L5 (-47, -21.6667) -> (-65, -21.6667)
  line L6 (-47, 47) -> (-47, -47)
extrude "Extrusion36" cut sketch "Skizze21" against normal blind 18 contours L0 L1 L3 L5 L6 | L1 L2 L3 L4 L6 bodies 1
extrude "Extrusion37" cut sketch "Skizze21" against normal blind 18 contours L1 L3 L4 L5 L6 bodies 3
ref_plane "Arbeitsebene4" through (106.1, -65.2765, -1.7101) normal (0, 0.939693, -0.34202) x (-1, 0, 0)
sketch "Skizze22" plane through (0, -57.091, 20.7794) normal (0, 0.939693, -0.34202) x (-1, 0, 0)
  line L0 (-84.6, -63.5816) -> (-84.6, -49.5816)
  line L1 (-84.6, -49.5816) -> (-70.6, -49.5816)
  line L2 (-70.6, -49.5816) -> (-70.6, -63.5816)
  line L3 (-70.6, -63.5816) -> (-84.6, -63.5816)
  line L4 (-160.6, -63.5816) -> (-160.6, -49.5816)
  line L5 (-160.6, -49.5816) -> (-146.6, -49.5816)
  line L6 (-146.6, -49.5816) -> (-146.6, -63.5816)
  line L7 (-146.6, -63.5816) -> (-160.6, -63.5816)
  line L8 (-141.6, -44.5816) -> (-141.6, -30.5816)
  line L9 (-141.6, -30.5816) -> (-127.6, -30.5816)
  line L10 (-127.6, -30.5816) -> (-127.6, -44.5816)
  line L11 (-127.6, -44.5816) -> (-141.6, -44.5816)
  line L12 (-65.6, -44.5816) -> (-65.6, -30.5816)
  line L13 (-65.6, -30.5816) -> (-51.6, -30.5816)
  line L14 (-51.6, -30.5816) -> (-51.6, -44.5816)
  line L15 (-51.6, -44.5816) -> (-65.6, -44.5816)
  line L16 (-70.6, -25.5816) -> (-84.6, -25.5816)
  line L17 (-84.6, -25.5816) -> (-84.6, -11.5816)
  line L18 (-84.6, -11.5816) -> (-70.6, -11.5816)
  line L19 (-70.6, -11.5816) -> (-70.6, -25.5816)
  line L20 (-160.6, -25.5816) -> (-160.6, -11.5816)
  line L21 (-160.6, -11.5816) -> (-146.6, -11.5816)
  line L22 (-146.6, -11.5816) -> (-146.6, -25.5816)
  line L23 (-146.6, -25.5816) -> (-160.6, -25.5816)
  line L24 (-127.6, -6.5816) -> (-141.6, -6.5816)
  line L25 (-141.6, -6.5816) -> (-141.6, 7.4184)
  line L26 (-141.6, 7.4184) -> (-127.6, 7.4184)
  line L27 (-127.6, 7.4184) -> (-127.6, -6.5816)
  line L28 (-65.6, -6.5816) -> (-65.6, 7.4184)
  line L29 (-65.6, 7.4184) -> (-51.6, 7.4184)
  line L30 (-51.6, 7.4184) -> (-51.6, -6.5816)
  line L31 (-51.6, -6.5816) -> (-65.6, -6.5816)
  line L32 (-70.6, -6.5816) -> (-84.6, -6.5816)
  line L33 (-84.6, -6.5816) -> (-84.6, 7.4184)
  line L34 (-84.6, 7.4184) -> (-70.6, 7.4184)
  line L35 (-70.6, 7.4184) -> (-70.6, -6.5816)
  line L36 (-160.6, -6.5816) -> (-160.6, 7.4184)
  line L37 (-160.6, 7.4184) -> (-146.6, 7.4184)
  line L38 (-146.6, 7.4184) -> (-146.6, -6.5816)
  line L39 (-146.6, -6.5816) -> (-160.6, -6.5816)
  line L40 (-127.6, -11.5816) -> (-127.6, -25.5816)
  line L41 (-127.6, -25.5816) -> (-141.6, -25.5816)
  line L42 (-141.6, -25.5816) -> (-141.6, -11.5816)
  line L43 (-141.6, -11.5816) -> (-127.6, -11.5816)
  line L44 (-65.6, -25.5816) -> (-65.6, -11.5816)
  line L45 (-65.6, -11.5816) -> (-51.6, -11.5816)
  line L46 (-51.6, -11.5816) -> (-51.6, -25.5816)
  line L47 (-51.6, -25.5816) -> (-65.6, -25.5816)
  line L48 (-70.6, -44.5816) -> (-84.6, -44.5816)
  line L49 (-84.6, -44.5816) -> (-84.6, -30.5816)
  line L50 (-84.6, -30.5816) -> (-70.6, -30.5816)
  line L51 (-70.6, -30.5816) -> (-70.6, -44.5816)
  line L52 (-160.6, -44.5816) -> (-160.6, -30.5816)
  line L53 (-160.6, -30.5816) -> (-146.6, -30.5816)
  line L54 (-146.6, -30.5816) -> (-146.6, -44.5816)
  line L55 (-146.6, -44.5816) -> (-160.6, -44.5816)
  line L56 (-127.6, -63.5816) -> (-141.6, -63.5816)
  line L57 (-141.6, -63.5816) -> (-141.6, -49.5816)
  line L58 (-141.6, -49.5816) -> (-127.6, -49.5816)
  line L59 (-127.6, -49.5816) -> (-127.6, -63.5816)
  line L60 (-65.6, -63.5816) -> (-65.6, -49.5816)
  line L61 (-65.6, -49.5816) -> (-51.6, -49.5816)
  line L62 (-51.6, -49.5816) -> (-51.6, -63.5816)
  line L63 (-51.6, -63.5816) -> (-65.6, -63.5816)
  line L64 (-103.6, -63.5816) -> (-103.6, -49.5816)
  line L65 (-103.6, -49.5816) -> (-89.6, -49.5816)
  line L66 (-89.6, -49.5816) -> (-89.6, -63.5816)
  line L67 (-89.6, -63.5816) -> (-103.6, -63.5816)
  line L68 (-179.6, -63.5816) -> (-179.6, -49.5816)
  line L69 (-179.6, -49.5816) -> (-165.6, -49.5816)
  line L70 (-165.6, -49.5816) -> (-165.6, -63.5816)
  line L71 (-165.6, -63.5816) -> (-179.6, -63.5816)
  line L72 (-122.6, -44.5816) -> (-122.6, -30.5816)
  line L73 (-122.6, -30.5816) -> (-108.6, -30.5816)
  line L74 (-108.6, -30.5816) -> (-108.6, -44.5816)
  line L75 (-108.6, -44.5816) -> (-122.6, -44.5816)
  line L76 (-46.6, -44.5816) -> (-46.6, -30.5816)
  line L77 (-46.6, -30.5816) -> (-32.6, -30.5816)
  line L78 (-32.6, -30.5816) -> (-32.6, -44.5816)
  line L79 (-32.6, -44.5816) -> (-46.6, -44.5816)
  line L80 (-103.6, -25.5816) -> (-103.6, -11.5816)
  line L81 (-103.6, -11.5816) -> (-89.6, -11.5816)
  line L82 (-89.6, -11.5816) -> (-89.6, -25.5816)
  line L83 (-89.6, -25.5816) -> (-103.6, -25.5816)
  line L84 (-179.6, -25.5816) -> (-179.6, -11.5816)
  line L85 (-179.6, -11.5816) -> (-165.6, -11.5816)
  line L86 (-165.6, -11.5816) -> (-165.6, -25.5816)
  line L87 (-165.6, -25.5816) -> (-179.6, -25.5816)
  line L88 (-122.6, -6.5816) -> (-122.6, 7.4184)
  line L89 (-122.6, 7.4184) -> (-108.6, 7.4184)
  line L90 (-108.6, 7.4184) -> (-108.6, -6.5816)
  line L91 (-108.6, -6.5816) -> (-122.6, -6.5816)
  line L92 (-46.6, -6.5816) -> (-46.6, 7.4184)
  line L93 (-46.6, 7.4184) -> (-32.6, 7.4184)
  line L94 (-32.6, 7.4184) -> (-32.6, -6.5816)
  line L95 (-32.6, -6.5816) -> (-46.6, -6.5816)
  line L96 (-103.6, -6.5816) -> (-103.6, 7.4184)
  line L97 (-103.6, 7.4184) -> (-89.6, 7.4184)
  line L98 (-89.6, 7.4184) -> (-89.6, -6.5816)
  line L99 (-89.6, -6.5816) -> (-103.6, -6.5816)
  line L100 (-165.6, -6.5816) -> (-179.6, -6.5816)
  line L101 (-179.6, -6.5816) -> (-179.6, 7.4184)
  line L102 (-179.6, 7.4184) -> (-165.6, 7.4184)
  line L103 (-165.6, 7.4184) -> (-165.6, -6.5816)
  line L104 (-122.6, -25.5816) -> (-122.6, -11.5816)
  line L105 (-122.6, -11.5816) -> (-108.6, -11.5816)
  line L106 (-108.6, -11.5816) -> (-108.6, -25.5816)
  line L107 (-108.6, -25.5816) -> (-122.6, -25.5816)
  line L108 (-46.6, -25.5816) -> (-46.6, -11.5816)
  line L109 (-46.6, -11.5816) -> (-32.6, -11.5816)
  line L110 (-32.6, -11.5816) -> (-32.6, -25.5816)
  line L111 (-32.6, -25.5816) -> (-46.6, -25.5816)
  line L112 (-103.6, -44.5816) -> (-103.6, -30.5816)
  line L113 (-103.6, -30.5816) -> (-89.6, -30.5816)
  line L114 (-89.6, -30.5816) -> (-89.6, -44.5816)
  line L115 (-89.6, -44.5816) -> (-103.6, -44.5816)
  line L116 (-179.6, -44.5816) -> (-179.6, -30.5816)
  line L117 (-179.6, -30.5816) -> (-165.6, -30.5816)
  line L118 (-165.6, -30.5816) -> (-165.6, -44.5816)
  line L119 (-165.6, -44.5816) -> (-179.6, -44.5816)
  line L120 (-122.6, -63.5816) -> (-122.6, -49.5816)
  line L121 (-122.6, -49.5816) -> (-108.6, -49.5816)
  line L122 (-108.6, -49.5816) -> (-108.6, -63.5816)
  line L123 (-108.6, -63.5816) -> (-122.6, -63.5816)
  line L124 (-46.6, -63.5816) -> (-46.6, -49.5816)
  line L125 (-46.6, -49.5816) -> (-32.6, -49.5816)
  line L126 (-32.6, -49.5816) -> (-32.6, -63.5816)
  line L127 (-32.6, -63.5816) -> (-46.6, -63.5816)
  line L128 (-18.2, -73.7492) -> (-18.2, 25.8835)
  line L129 (-18.2, 25.8835) -> (-194, 25.8835)
  line L130 (-194, 25.8835) -> (-194, -73.7492)
  line L131 (-194, -73.7492) -> (-18.2, -73.7492)
  line L132 (-186.6, 18.0671) -> (-25.6, 18.0671)
  line L133 (-25.6, 18.0671) -> (-25.6, -65.9329)
  line L134 (-25.6, -65.9329) -> (-186.6, -65.9329)
  line L135 (-186.6, -65.9329) -> (-186.6, 18.0671)
  circle A0 centre (-39.6, 0.4184) radius 2
  circle A1 centre (-58.6, 0.4184) radius 2
  circle A2 centre (-77.6, 0.4184) radius 2
  circle A3 centre (-96.6, 0.4184) radius 2
  circle A4 centre (-115.6, 0.4184) radius 2
  circle A5 centre (-134.6, 0.4184) radius 2
  circle A6 centre (-153.6, 0.4184) radius 2
  circle A7 centre (-172.6, 0.4184) radius 2
  circle A8 centre (-39.6, -18.5816) radius 2
  circle A9 centre (-58.6, -18.5816) radius 2
  circle A10 centre (-77.6, -18.5816) radius 2
  circle A11 centre (-96.6, -18.5816) radius 2
  circle A12 centre (-115.6, -18.5816) radius 2
  circle A13 centre (-134.6, -18.5816) radius 2
  circle A14 centre (-153.6, -18.5816) radius 2
  circle A15 centre (-172.6, -18.5816) radius 2
  circle A16 centre (-39.6, -37.5816) radius 2
  circle A17 centre (-58.6, -37.5816) radius 2
  circle A18 centre (-77.6, -37.5816) radius 2
  circle A19 centre (-96.6, -37.5816) radius 2
  circle A20 centre (-115.6, -37.5816) radius 2
  circle A21 centre (-134.6, -37.5816) radius 2
  circle A22 centre (-153.6, -37.5816) radius 2
  circle A23 centre (-172.6, -37.5816) radius 2
  circle A24 centre (-39.6, -56.5816) radius 2
  circle A25 centre (-58.6, -56.5816) radius 2
  circle A26 centre (-77.6, -56.5816) radius 2
  circle A27 centre (-96.6, -56.5816) radius 2
  circle A28 centre (-115.6, -56.5816) radius 2
  circle A29 centre (-134.6, -56.5816) radius 2
  circle A30 centre (-153.6, -56.5816) radius 2
  circle A31 centre (-172.6, -56.5816) radius 2
  point P0 (-194, -23.9329)
  point P1 (-106.1, 25.8835)
  point P2 (-106.1, 18.0671)
  point P3 (-186.6, -23.9329)
  dimension "d183" = 4
  dimension "d186" = -19
  dimension "d187" = -19
  dimension "d189" = 161
  dimension "d190" = 84
  constraint horizontal L132
  constraint vertical L133
  constraint horizontal L134
  constraint vertical L135
  constraint midpoint L130 P0
  constraint midpoint L129 P1
  constraint midpoint L132 P2
  constraint midpoint L135 P3
  constraint vertical P1 P2
  constraint horizontal P0 P3
  measures "d183" diameter of A0
  measures "d189" distance of L133.end L134.end
  measures "d190" distance of L132.start L134.end
extrude "Extrusion38" add sketch "Skizze22" along normal blind 1.6 separate body contours L0 L1 L2 L3 | L4 L5 L6 L7 | L8 L9 L10 L11 | L12 L13 L14 L15 | L16 L17 L18 L19 | L20 L21 L22 L23 | L24 L25 L26 L27 | L28 L29 L30 L31 | L32 L33 L34 L35 | L36 L37 L38 L39 | L40 L41 L42 L43 | L44 L45 L46 L47 | L48 L49 L50 L51 | L52 L53 L54 L55 | L56 L57 L58 L59 | L60 L61 L62 L63 | L64 L65 L66 L67 | L68 L69 L70 L71 | L72 L73 L74 L75 | L76 L77 L78 L79 | L80 L81 L82 L83 | L84 L85 L86 L87 | L88 L89 L90 L91 | L92 L93 L94 L95 | L96 L97 L98 L99 | L100 L101 L102 L103 | L104 L105 L106 L107 | L108 L109 L110 L111 | L112 L113 L114 L115 | L116 L117 L118 L119 | L120 L121 L122 L123 | L124 L125 L126 L127 | L132 L133 L134 L135 makes body 15
sketch "Skizze23" plane through (0, -55.5875, 20.2322) normal (0, 0.939693, -0.34202) x (-1, 0, 0)
  circle A0 centre (-77.6, -56.5816) radius 2
  circle A1 centre (-96.6, -56.5816) radius 2
  circle A2 centre (-172.6, -56.5816) radius 2
  circle A3 centre (-115.6, -56.5816) radius 2
  circle A4 centre (-134.6, -56.5816) radius 2
  circle A5 centre (-153.6, -56.5816) radius 2
  circle A6 centre (-39.6, -56.5816) radius 2
  circle A7 centre (-153.6, -18.5816) radius 2
  circle A8 centre (-77.6, -37.5816) radius 2
  circle A9 centre (-172.6, -37.5816) radius 2
  circle A10 centre (-96.6, -37.5816) radius 2
  circle A11 centre (-115.6, -37.5816) radius 2
  circle A12 centre (-58.6, -37.5816) radius 2
  circle A13 centre (-39.6, -37.5816) radius 2
  circle A14 centre (-134.6, -37.5816) radius 2
  circle A15 centre (-172.6, -18.5816) radius 2
  circle A16 centre (-58.6, -56.5816) radius 2
  circle A17 centre (-153.6, -37.5816) radius 2
  circle A18 centre (-134.6, -18.5816) radius 2
  circle A19 centre (-115.6, -18.5816) radius 2
  circle A20 centre (-96.6, -18.5816) radius 2
  circle A21 centre (-77.6, -18.5816) radius 2
  circle A22 centre (-58.6, -18.5816) radius 2
  circle A23 centre (-39.6, -18.5816) radius 2
  circle A24 centre (-172.6, 0.4184) radius 2
  circle A25 centre (-153.6, 0.4184) radius 2
  circle A26 centre (-134.6, 0.4184) radius 2
  circle A27 centre (-115.6, 0.4184) radius 2
  circle A28 centre (-96.6, 0.4184) radius 2
  circle A29 centre (-77.6, 0.4184) radius 2
  circle A30 centre (-58.6, 0.4184) radius 2
  circle A31 centre (-39.6, 0.4184) radius 2
  line L0 (-186.6, -65.9329) -> (-25.6, -65.9329)
  line L1 (-25.6, -65.9329) -> (-25.6, 18.0671)
  line L2 (-25.6, 18.0671) -> (-186.6, 18.0671)
  line L3 (-186.6, 18.0671) -> (-186.6, -65.9329)
  line L4 (-186.6, 18.0671) -> (-25.6, 18.0671)
  point P0 (-39.6, 0.4184)
  dimension "d188" = 25
sketch "Skizze26" plane through (0, 0, 65) normal (0, 0, 1) x (-1, 0, 0)
  line L0 (-187.7, 41.4485) -> (-152.7, 41.4485)
  line L1 (-152.7, 41.4485) -> (-152.7, 15.4485)
  line L2 (-152.7, 15.4485) -> (-187.7, 15.4485)
  line L3 (-187.7, 15.4485) -> (-187.7, 41.4485)
  circle A0 centre (-187.7, 28.4485) radius 1.6
  circle A1 centre (-152.7, 28.4485) radius 1.6
  circle A2 centre (-172.2, 27.5985) radius 7
  line L4 (-212.2, 17.299) -> (-212.2, 58.4485)
  line L5 (-212.2, 58.4485) -> (-194.2, 58.4485)
  dimension "d201" = 35
  dimension "d202" = 26
  dimension "d203" = 3.2
  dimension "d204" = 3.2
  dimension "d205" = 14
  dimension "d260" = 13.85
  constraint horizontal L0
  constraint vertical L1
  constraint horizontal L2
  constraint vertical L3
  constraint midpoint L3 A0.centre
  constraint midpoint L1 A1.centre
  measures "d201" distance of L0.start L0.end
  measures "d202" distance of L0.start L2.end
  measures "d203" diameter of A0
  measures "d204" diameter of A1
  measures "d205" diameter of A2
  measures "d260" distance of L0 A2.centre
extrude "Extrusion40" cut sketch "Skizze26" against normal up to surface (18 mm away) contours L3 A0 | L3 A0 | L1 A1 | L1 A1 | A2 bodies 4